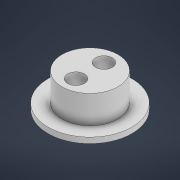
# Autodesk Inventor part: InputShaft3
Saved by Autodesk Inventor 2021 (Build 250183000, 183)
## iProperties
Created: 2022-10-09
Part Number: InputShaft3
Material: Ogólny
Document SubType Name: Modeling
Designer: MicnedSQ
Density: 1 g/cm^3
Appearance: Domyślna
Author: MicnedSQ
Autodesk Inventor part; units mm, degrees
ref_plane "YZ Plane" through (0, 0, 0) normal (1, 0, 0) x (0, 1, 0)
ref_plane "XZ Plane" through (0, 0, 0) normal (0, 1, 0) x (-1, 0, 0)
ref_plane "XY Plane" through (0, 0, 0) normal (0, 0, 1) x (1, 0, 0)
sketch "Szkic1" plane through (0, 0, 0) normal (0, 1, 0) x (-1, 0, 0)
  circle A0 centre (0, 0) radius 7.5
  dimension "d0" = 15
  constraints: 1 centre point, 1 coincident
  measures "d0" diameter of A0
extrude "Wyciągnięcie proste1" add sketch "Szkic1" along normal blind 1
sketch "Szkic2" plane through (0, 1, 0) normal (0, 1, 0) x (1, 0, 0)
  circle A0 centre (0, 0) radius 5
  dimension "d3" = 10
  constraints: 1 centre point, 1 coincident
  measures "d3" diameter of A0
extrude "Wyciągnięcie proste2" add sketch "Szkic2" along normal blind 5
sketch "Szkic3" plane through (0, 6, 0) normal (0, 1, 0) x (1, 0, 0)
  circle A0 centre (0, -2.5) radius 1.5
  point P0 (0, 0)
  dimension "d6" = 3
  dimension "d7" = 2.5
  constraints: 1 centre point
  measures "d6" diameter of A0
  measures "d7" distance of point (0, 0) A0.centre
extrude "Wyciągnięcie proste3" cut sketch "Szkic3" against normal up to surface (6 mm away)
mirror "Odbij2" about plane through (0, 0, 0) normal (0, 0, 1) of "Wyciągnięcie proste3"
